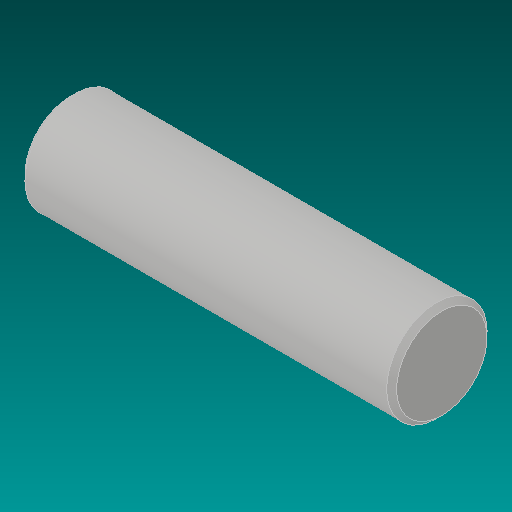
# Autodesk Inventor part: NSFMR10-37(000_000)_s
Saved by Autodesk Inventor 2020 (Build 240168000, 168)
## iProperties
Created: 2022-11-16
Part Number: NSFMR10-37(000_000)_s
Material: Generic
Catalog Web Link: www.cadenas.de
Description: NSFMR, SFMR, PSFMR, SSFMR, SSSFMR, NSFHR, SFHR, PSFHR, PPSFHR SSFHR, SSSFHR, NSFR, SFR, PSFR, PPSFR, SSFR, SSSFR, HFR, PHFR_shaft-Rotary Shafts - Straight -
Vendor: MISUMI
Document SubType Name: Modeling
Designer: psAdmin
Manufacturer: MISUMI
Mass: 2.89838 g
Surface Area: 13.0042 cm^2
Volume: 2.89838 cm^3
Density: 1 g/cm^3
Appearance: PSOLRGB-175-175-175
Category: PARTsolutions
Company: MISUMI
PSOL_IDENT_0: {$CADENAS_DATA/23d-libs/misumi/metric/11_rotary_shafts/11_components/psfr/psfr.prj},560 {VTYP=3D},{N
PSOL_IDENT_1: B=NSFMR10-37(000_000)_s},{LINA=NSFMR10-37},{NN=NSFMR, SFMR, PSFMR, SSFMR, SSSFMR, NSFHR, SFHR, PSFHR
PSOL_IDENT_2: , PPSFHR SSFHR, SSSFHR, NSFR, SFR, PSFR, PPSFR, SSFR, SSSFR, HFR, PHFR_shaft},{DATE=21.04.2022 07:40
PSOL_IDENT_3: :10},{GEOMDATE=27.07.2021 07:07:13},{VERSION=},{LINEID=30},{WBVAR=TS,MAT,ST,ALT1,L,ALT2,KC,A,WKC,C,K
PSOL_IDENT_4: ,E,KZ,Z,ALT3,FC,GALT3,WFC,J,WALT3,V,ALT4,SFC,SG,AG,ALT10,KWC,ALT11,WC,ALT6,TA,TB,ALT5,UC,ALT7,SC,ALT
PSOL_IDENT_5: 32,CD,ALT34,TCJ,WTCJ,XT,HCJ,WHCJ,XH},{WBNUMERIC=L,KC,A,WKC,C,K,E,KZ,Z,FC,GALT3,WFC,J,WALT3,V,SFC,SG,
PSOL_IDENT_6: AG,KWC,WC,TA,TB,UC,SC,TCJ,WTCJ,XT,HCJ,WHCJ,XH}  {NB=NSFMR10-37(000_000)_s},{LINA=NSFMR10-37},{KT=DUM
PSOL_IDENT_7: MY},{PN=NSFMR10-37},{TYPE=NSFMR},{TS=M},{TSALG= 'M','h9 (Cold-drawn)','H','h7 (Ground)','','g6 (Grou
PSOL_IDENT_8: nd)' },{MAT=S45C},{MATALG= 'S45C','S45C Equivalent', 'SUS304','304 Stainless Steel' },{ST=},{STALG= ''
PSOL_IDENT_9: ,'-','BO','Black Oxide', 'ENP','Electroless Nickel Plating' },{D=10.0},{ALT1=},{L=37.0},{LALG=[15:80
PSOL_IDENT_10: 0/0.1]},{LMIN=15},{LMAX=800},{NOTE=Not Applicable},{ALT2=},{ALT2ALG= '', 'w/o Key Grooves','KC','wit
PSOL_IDENT_11: h KC (Key Groove)','WKC','with WKC (Two Key Grooves)','KCWKC','with KC + WKC (Three Key Grooves)','K
PSOL_IDENT_12: Z','with KC + WKC + KZ (Four Key Grooves)' },{ALT2PN=},{KC=0.0},{KCALG=[0]},{KCMIN=0},{KCMAX=0},{A=0
PSOL_IDENT_13: .0},{AALG=[0]},{AMIN=3},{AMAX=0},{WKC=0.0},{WKCALG=[0]},{WKCMIN=0},{WKCMAX=0},{C=0.0},{CALG=[0]},{CM
PSOL_IDENT_14: IN=3},{CMAX=0},{K=0.0},{KALG=[0]},{KMIN=0},{KMAX=32},{E=0.0},{EALG=[0]},{EMIN=3},{EMAX=35},{KZ=0.0},
PSOL_IDENT_15: {KZALG=[0]},{KZMIN=39},{KZMAX=34},{Z=0.0},{ZALG=[0]},{ZMIN=3},{ZMAX=37},{CIFKC=1},{CIFWKC=1},{CIFK=1
PSOL_IDENT_16: },{CIFKZ=2},{PCUT3D=0.000},{QCUT3D=0},{BB=3},{BBALT2=3},{TT=1.8},{TTALT2=1.8},{ALT3=},{ALT3ALG= '', '
PSOL_IDENT_17: w/o Set Screw Flat','FC','with FC (Adds a Set Screw Flat)','WFC','with WFC (Adds Two Set Screw Flats
PSOL_IDENT_18: )','FCWFC','with FC + WFC (Adds Three Set Screw Flats)' },{ALT3PN=},{FC=0},{FCALG=[0]},{FCMIN=0},{FC
PSOL_IDENT_19: MAX=36},{GALT3=0},{GALT3ALG=[0]},{GALT3MIN=1},{GALT3MAX=37},{GALT3MAX2=31},{GALT3MAX3=34},{WFC=0},{W
PSOL_IDENT_20: FCALG=[0]},{WFCMIN=0},{WFCMIN2=2},{WFCMAX=33},{WFCMAX2=-3},{WFCMAX3=-4},{J=0},{JALG=[0]},{JMIN=1},{J
PSOL_IDENT_21: MAX=34},{JMAX2=-2},{JMAX3=-5},{WALT3=0},{WALT3ALG=[0]},{WALT3MIN=0},{WALT3MIN2=39},{WALT3MAX=34},{WA
PSOL_IDENT_22: LT3MAX2=34},{WALT3MAX3=34},{V=0},{VALG=[0]},{VMIN=1},{VMAX=35},{VMAX2=35},{VMAX3=35},{CIFFC=0},{ALT4=
PSOL_IDENT_23: },{ALT4ALG= '', 'w/o SFC (2 Set Screw Flats (Angle Specified))', 'SFC'  , 'with SFC (2 Set Screw Fla
PSOL_IDENT_24: ts (Angle Specified))'},{ALT4PN=},{SFC=0},{SFCALG=[0]},{SFCMIN=0},{SFCMAX=36},{SG=0},{SGALG=[0]},{SG
PSOL_IDENT_25: MIN=1},{SGMAX=37},{AG=0},{AGALG=[0]},{H=0.0},{CIFSFC=0},{ALT10=},{ALT10ALG= '', 'w/o KWC (2 Set Scre
PSOL_IDENT_26: w Flats at both ends)', 'KWC', 'with KWC (2 Set Screw Flats at both ends)' },{ALT10PN=},{KWC=0},{KWC
PSOL_IDENT_27: ALG=[0]},{KWCMIN=1},{KWCMAX=17.5},{WALT10=8},{ALT11=},{ALT11ALG= '','Not applicable' },{ALT11PN=},{W
PSOL_IDENT_28: C=0.0},{WCALG=[0]},{ALT6=},{ALT6ALG= '','w/o Retaining Ring Groove','TA','with TA (Retaining Ring Gr
PSOL_IDENT_29: oove)','TB','with TB (Retaining Ring Groove)','TATB','with TA + TB (Two Retaining Ring Grooves)' },{
PSOL_IDENT_30: ALT6PN=},{TA=0.0},{TAALG=[0]},{TAMIN=2},{TAMAX=0},{TB=0.0},{TBALG=[0]},{TBMIN=2},{TBMAX=0},{DDALT6=0
PSOL_IDENT_31: .0},{MM=0.00},{ALT5=},{ALT5ALG= '', 'w/o UC (Slit Cam Groove)', 'UC', 'with UC (Slit Cam Groove)'},{
PSOL_IDENT_32: ALT5PN=},{UC=0},{UCALG=[0]},{UCMIN=1},{UCMAX=31},{DDALT5=0},{LL1=0},{ALT7=},{ALT7ALG= '', 'w/o SC (W
PSOL_IDENT_33: rench Flats)', 'SC', 'with SC (Wrench Flats)'},{ALT7PN=},{SC=0},{SCALG=[0]},{SCMIN=0},{SCMAX=29},{WA
PSOL_IDENT_34: LT7=0},{LL2=0},{LL2ALG=8},{CIFSC=0},{ALT32=},{ALT32ALG=  '','w/o CD (Changes Part D Chamfering)','-C
PSOL_IDENT_35: D', 'with CD (Changes Part D Chamfering)' },{ALT32PN=},{CD=},{CDALG= '','N/A' },{CD3D=0.5},{CIF32=0}
PSOL_IDENT_36: ,{CIF320=0},{CIFTA=0},{CIFTB=0},{ERRORPN=},{ERRORALT23=OK},{ERRORALT24=OK},{ERRORALT25=OK},{ERRORALT
PSOL_IDENT_37: 26=OK},{ERRORALT27=OK},{ERRORALT210=OK},{ERRORALT34=OK},{ERRORALT35=OK},{ERRORALT36=OK},{ERRORALT37=
PSOL_IDENT_38: OK},{ERRORALT310=OK},{ERRORALT45=OK},{ERRORALT46=OK},{ERRORALT47=OK},{ERRORALT410=OK},{ERRORALT56=OK
PSOL_IDENT_39: },{ERRORALT57=OK},{ERRORALT510=OK},{ERRORALT610=OK},{ERRORALT75=OK},{ERRORALT76=OK},{ERRORALT710=OK}
PSOL_IDENT_40: ,{ALT34=},{ALT34ALG= '','Not applicable'},{TCJ=0},{WTCJ=0},{XT=0},{TM=4},{TCJALG=[0]},{TCJMIN=0.000}
PSOL_IDENT_41: ,{TCJMAX=15.000},{TCJMAX1=15.000},{HCJ=0},{WHCJ=0},{XH=0},{HP=4},{HCJALG=[0]},{HCJMIN=0.000},{HCJMAX=
PSOL_IDENT_42: 15.000},{HCJMAX1=15.000},{LCJ=0},{LMINX=15},{XCJMIN=4.000},{XALG=[0]},{XCJMAX=15.000},{WHCJMIN=0.000
PSOL_IDENT_43: },{WTCJMIN=0.000},{WTCJALG=[0]},{WHCJALG=[0]},{XHCJMIN=4.000},{XHALG=[0]}
NB: NSFMR10-37(000_000)_s
NN: NSFMR, SFMR, PSFMR, SSFMR, SSSFMR, NSFHR, SFHR, PSFHR, PPSFHR SSFHR, SSSFHR, NSFR, SFR, PSFR, PPSFR, SSFR, SSSFR, HFR, PHFR_shaft
NT: Rotary Shafts - Straight -
NBSYN: $PN.($ALT34.$TCJ.$WTCJ.$XT._$HCJ.$WHCJ.$XH.)_s
LINA: NSFMR10-37
CATALOG: Misumi
PN: NSFMR10-37
TS: h9 (Cold-drawn)
MAT: S45C Equivalent
ST: -
D: 10
ALT1: w/o LKC (Changes L Tolerance)
L: 37
ALT2: w/o Key Grooves
KC: 0
A: 0
WKC: 0
C: 0
K: 0
E: 0
KZ: 0
Z: 0
ALT3: w/o Set Screw Flat
FC: 0
GALT3: 0
WFC: 0
J: 0
WALT3: 0
V: 0
ALT4: w/o SFC (2 Set Screw Flats (Angle Specified))
SFC: 0
SG: 0
AG: 0
H: 0
ALT10: w/o KWC (2 Set Screw Flats at both ends)
KWC: 0
ALT11: Not applicable
WC: 0
ALT6: w/o Retaining Ring Groove
TA: 0
TB: 0
DDALT6: 0
MM: 0
ALT5: w/o UC (Slit Cam Groove)
UC: 0
DDALT5: 0
LL1: 0
ALT7: w/o SC (Wrench Flats)
SC: 0
WALT7: 0
LL2: 0
ALT32: w/o CD (Changes Part D Chamfering)
CD: N/A
ALT34: Not applicable
TCJ: 0
WTCJ: 0
XT: 0
HCJ: 0
WHCJ: 0
XH: 0
SUPPLIER: MISUMI
ARTICLENO: NSFMR10-37(000_000)_s
BOMINFO: NSFMR10-37
CREATOR: CADENAS GmbH
d1: 0.000 mm
Title: NSFMR10-37
Author: Cadenas PARTsolutions
Comments: Rotary Shafts - Straight -
Autodesk Inventor part; units mm, degrees
sketch "Sketch_1" plane through (0, 0, 0) normal (0, 0, 1) x (1, 0, 0)
  line L0 (37, 0) -> (0, 0)
  line L1 (0, 0) -> (0, 4.5)
  line L2 (0, 4.5) -> (0.5, 5)
  line L3 (0.5, 5) -> (36.5, 5)
  line L4 (36.5, 5) -> (37, 4.5)
  line L5 (37, 4.5) -> (37, 0)
  line L6 (37, 0) -> (0, 0)
  constraints: 14 end point
revolve "Revolution1" add sketch "Sketch_1" angle 360 about axis through (37, 0, 0) along (1, 0, 0)
ref_plane "COMBINATION_MODULE_XY" through (0, 0, 0) normal (1, 0, 0) x (0, 0, -1)
ref_plane "COMBINATION_MODULE_YZ" through (0, 0, 0) normal (0, 0, -1) x (0, 1, 0)
ref_plane "COMBINATION_MODULE_ZX" through (0, 0, 0) normal (0, 1, 0) x (1, 0, 0)
body "Solid1"
